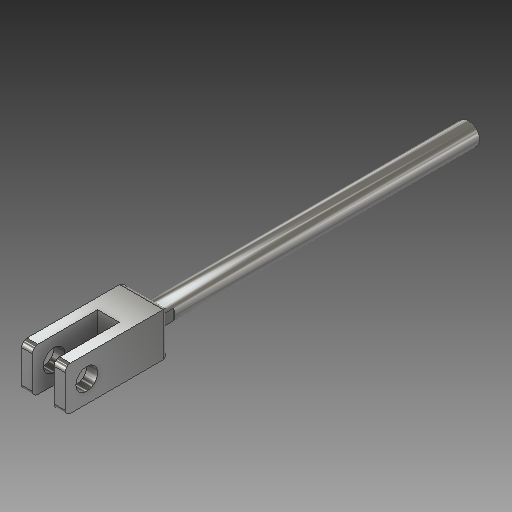
# Autodesk Inventor part: cylinder piston
Saved by Autodesk Inventor 2017 SP1 (Build 210196100, 196)
## iProperties
Created: 2018-01-27
Part Number: cylinder piston
Material: Generic
Document SubType Name: Modeling
Designer: Ben
Density: 1 g/cm^3
Appearance: Chrome - Polished
Mass: 6.07195 g
Surface Area: 39.2792 cm^2
Volume: 6.07195 cm^3
Author: Ben
Autodesk Inventor part; units mm, degrees
ref_plane "YZ Plane" through (0, 0, 0) normal (1, 0, 0) x (0, 1, 0)
ref_plane "XZ Plane" through (0, 0, 0) normal (0, 1, 0) x (-1, 0, 0)
ref_plane "XY Plane" through (0, 0, 0) normal (0, 0, 1) x (1, 0, 0)
sketch "Sketch1" plane through (0, 0, 0) normal (0, 0, 1) x (1, 0, 0)
  circle A0 centre (0, 0) radius 3.175
  dimension "d0" = 6.35
  constraints: 1 centre point, 1 coincident
  measures "d0" diameter of A0
extrude "Extrusion1" add sketch "Sketch1" along normal blind 88.9
sketch "Sketch2" plane through (0, 0, 88.9) normal (0, 0, 1) x (1, 0, 0)
  circle A0 centre (0, 0) radius 3.175 projected
  arc A1 (2.7496, 1.5875) -> (-2.7496, 1.5875) centre (0, 0) ccw
  arc A2 (-2.7496, -1.5875) -> (2.7496, -1.5875) centre (0, 0) ccw
  line L0 (2.7496, 1.5875) -> (2.7496, -1.5875)
  line L1 (-2.7496, 1.5875) -> (-2.7496, -1.5875)
  line L2 (0, 3.175) -> (0, -3.175) construction
  dimension "d3" = 3.175
  constraints: 8 point on circle, 6 end point, 3 coincident, 2 centre point, 1 concentric, 1 midpoint, 1 parallel, 1 vertical
  measures "d3" distance of L0.start L0.end
extrude "Extrusion2" add sketch "Sketch2" along normal blind 5.08 contours L0 A0 L1
sketch "Sketch3" plane through (0, 0, 93.98) normal (0, 0, 1) x (1, 0, 0)
  line L0 (-6.35, -6.35) -> (6.35, -6.35)
  line L1 (6.35, -6.35) -> (6.35, 6.35)
  line L2 (6.35, 6.35) -> (-6.35, 6.35)
  line L3 (-6.35, 6.35) -> (-6.35, -6.35)
  line L4 (-6.35, -6.35) -> (6.35, 6.35) construction
  line L5 (6.35, -6.35) -> (-6.35, 6.35) construction
  point P0 (0, 0)
  dimension "d6" = 12.7
  constraints: 12 end point, 2 midpoint, 2 parallel, 2 perpendicular, 1 horizontal
  measures "d6" distance of L2.end L1.end
extrude "Extrusion3" add sketch "Sketch3" along normal blind 11.176
sketch "Sketch4" plane through (0, 0, 105.156) normal (0, 0, 1) x (1, 0, 0)
  line L0 (6.35, 6.35) -> (-6.35, 6.35) projected
  line L1 (-6.35, -6.35) -> (6.35, -6.35) projected
  line L2 (6.35, 6.35) -> (3.175, 6.35)
  line L3 (3.175, 6.35) -> (3.175, -6.35)
  line L4 (3.175, -6.35) -> (6.35, -6.35)
  line L5 (6.35, -6.35) -> (6.35, 6.35)
  line L6 (-6.35, 6.35) -> (-3.175, 6.35)
  line L7 (-3.175, 6.35) -> (-3.175, -6.35)
  line L8 (-3.175, -6.35) -> (-6.35, -6.35)
  line L9 (-6.35, -6.35) -> (-6.35, 6.35)
  line L10 (3.175, 0) -> (-3.175, 0) construction
  point P0 (0, 0)
  point P1 (0, 0)
  dimension "d9" = 6.35
  constraints: 18 end point, 4 parallel, 3 midpoint, 3 point on line, 2 horizontal, 2 perpendicular, 1 coincident
  measures "d9" distance of L10.start L10.end
extrude "Extrusion4" add sketch "Sketch4" along normal blind 19.05 contours L5 L1 L3 L0 | L7 L1 L9 L0
sketch "Sketch5" plane through (6.35, -6.35, 93.98) normal (1, 0, 0) x (0, 0, -1)
  line L0 (-30.226, 12.7) -> (-30.226, 0) construction
  line L1 (-30.226, 6.35) -> (-23.876, 6.35) construction
  circle A0 centre (-23.876, 6.35) radius 3.175
  point P0 (93.98, 6.35)
  dimension "d12" = 6.35
  dimension "d13" = 6.35
  constraints: 2 end point, 1 centre point, 1 coincident, 1 horizontal, 1 midpoint
  measures "d12" diameter of A0
  measures "d13" distance of L1.start L1.end
extrude "Extrusion5" cut sketch "Sketch5" against normal through all
fillet "Fillet1" radius 1.5875 8 edges at (4.7625, 6.35, 124.206) (4.7625, -6.35, 124.206) (-4.7625, -6.35, 124.206) (-4.7625, 6.35, 124.206) (6.35, 0, 93.98) (0, 6.35, 93.98) (-6.35, 0, 93.98) (0, -6.35, 93.98)
body "Solid1"
